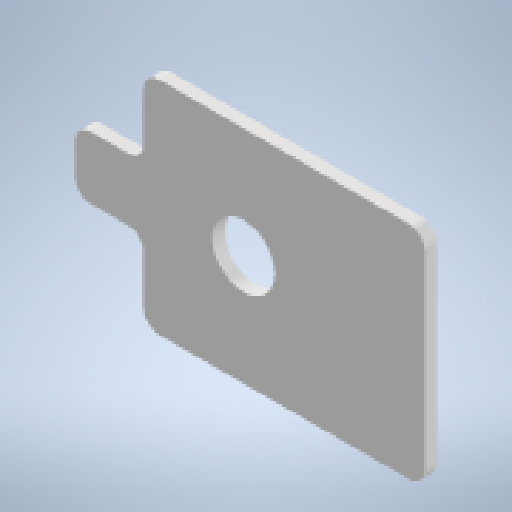
# Autodesk Inventor part: plate_3
Saved by Autodesk Inventor 2024 (Build 280153000, 153)
## iProperties
Created: 2026-02-08
Part Number: plate_3
Material: Generic
Document SubType Name: Modeling
Designer: SEMEN
Density: 1 g/cm^3
Appearance: Default
Author: SEMEN
Autodesk Inventor part; units mm, degrees
ref_plane "YZ Plane" through (0, 0, 0) normal (1, 0, 0) x (0, 1, 0)
ref_plane "XZ Plane" through (0, 0, 0) normal (0, 1, 0) x (-1, 0, 0)
ref_plane "XY Plane" through (0, 0, 0) normal (0, 0, 1) x (1, 0, 0)
sketch "Sketch1" plane through (0, 0, 0) normal (0, 0, 1) x (1, 0, 0)
  circle A0 centre (13.407, 27.6606) radius 2.5 construction
  circle A1 centre (13.407, 27.6606) radius 10 construction
  circle A2 centre (57.407, 53.064) radius 2.5 construction
  circle A3 centre (57.407, 53.064) radius 10 construction
  circle A4 centre (57.407, 2.2572) radius 2.5 construction
  circle A5 centre (57.407, 2.2572) radius 10 construction
  line L0 (125.407, 63.064) -> (125.407, -7.7428)
  line L1 (125.407, -7.7428) -> (25.407, -7.7428)
  line L2 (125.407, 82.5038) -> (125.407, 159.5038) projected
  line L3 (57.407, 53.064) -> (57.407, 2.2572) construction
  circle A6 centre (57.407, 27.6606) radius 10
  line L4 (47.1446, 17.3983) -> (70.9177, 41.1714) construction
  circle A7 centre (47.5075, 17.7611) radius 4 construction
  circle A8 centre (67.3065, 37.5601) radius 4 construction
  line L5 (45.5703, 39.4972) -> (72.2419, 12.8257) construction
  circle A9 centre (47.5075, 37.5601) radius 4 construction
  circle A10 centre (67.3065, 17.7611) radius 4 construction
  line L6 (25.407, -109.9962) -> (25.407, 140.0038) projected
  line L7 (3.407, 37.6606) -> (25.407, 37.6606)
  line L8 (3.407, 17.6606) -> (25.407, 17.6606)
  line L9 (25.407, 63.064) -> (125.407, 63.064)
  line L10 (3.407, 17.6606) -> (3.407, 37.6606)
  point P0 (0, 0)
  point P1 (57.407, 63.064)
  point P2 (13.407, 37.6606)
  point P3 (13.407, 17.6606)
  point P4 (57.407, -7.7428)
  dimension "d1" = 20
  dimension "d2" = 45
  dimension "d3" = 8
  dimension "d4" = 8
  dimension "d5" = 45
  dimension "d6" = 8
  dimension "d7" = 8
  constraints: 18 end point, 10 point on line, 9 tangent, 5 centre point, 4 coincident, 3 perpendicular, 2 parallel, 1 collinear, 1 horizontal, 1 midpoint, 1 vertical
  measures "d1" diameter of A6
  measures "d2" angle of L3 L4
  measures "d3" diameter of A7
  measures "d4" diameter of A8
  measures "d5" angle of L3 L5
  measures "d6" diameter of A9
  measures "d7" diameter of A10
extrude "Extrusion1" add sketch "Sketch1" along normal blind 4
fillet "Fillet1" radius 5 8 edges at (25.407, -7.7428, 2) (25.407, 63.064, 2) (125.407, 63.064, 2) (125.407, -7.7428, 2) (3.407, 17.6606, 2) (3.407, 37.6606, 2) (25.407, 17.6606, 2) (25.407, 37.6606, 2)
hole "Hole1" at (67.3065, 37.5601, 0) at (47.5075, 37.5601, 0) at (47.5075, 17.7611, 0) at (67.3065, 17.7611, 0) direction (0, 0, 1) diameter 3.4 end through all countersink diameter 6.6 countersink angle 90 clearance for "Countersunk Head GOST 12876-67" size "M3" standard "GOST"
sketch "Sketch2" plane through (0, 0, 4) normal (0, 0, 1) x (1, 0, 0)
  circle A0 centre (13.407, 27.6606) radius 2.5 projected
  circle A1 centre (57.407, 2.2572) radius 2.5 projected
  circle A2 centre (57.407, 53.064) radius 2.5 projected
  line L0 (10.407, 27.6606) -> (16.407, 27.6606) construction
  line L1 (10.407, 24.9106) -> (16.407, 24.9106)
  line L2 (16.407, 30.4106) -> (10.407, 30.4106)
  arc A3 (10.407, 30.4106) -> (10.407, 24.9106) centre (10.407, 27.6606) ccw
  arc A4 (16.407, 24.9106) -> (16.407, 30.4106) centre (16.407, 27.6606) ccw
  point P0 (0, 0)
  dimension "d25" = 3
  dimension "d26" = 5.5
  constraints: 8 end point, 4 point on circle, 4 tangent, 2 centre point, 1 horizontal, 1 midpoint, 1 parallel
  measures "d25" distance of A0.centre L0.end
  measures "d26" diameter of A4
hole "Hole2" at (57.407, 53.064, 4) at (57.407, 2.2572, 4) direction (0, 0, -1) diameter 5.5 end through all countersink diameter 10.4 countersink angle 90 clearance for "Countersunk Head GOST 12876-67" size "M5" standard "GOST"
sketch "Sketch3" plane through (0, 0, 4) normal (0, 0, 1) x (1, 0, 0)
  arc A0 (10.407, 30.4106) -> (10.407, 24.9106) centre (10.407, 27.6606) ccw projected
  line L0 (16.407, 30.4106) -> (10.407, 30.4106) projected
  line L1 (10.407, 24.9106) -> (16.407, 24.9106) projected
  arc A1 (16.407, 24.9106) -> (16.407, 30.4106) centre (16.407, 27.6606) ccw projected
  point P0 (0, 0)
extrude "Extrusion2" cut sketch "Sketch3" against normal up to surface (4 mm away)
body "Solid1"
